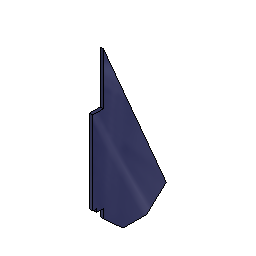
FIN_BUILD_1 (Autodesk Fusion 360 design; units mm, degrees)
Autodesk Fusion 360 part; units mm, degrees
note: some values were not read from the file. Set by a fixed rule: which sketch regions a step uses.
sketch "Sketch1" plane through (0, 0, 0) normal (0, 0, 1) x (1, 0, 0)
  circle A0 centre (0, 0) radius 29.75
  circle A1 centre (0, 0) radius 14.45
  circle A2 centre (0, 0) radius 18.45
  line L0 (0, 0) -> (0, 29.75) construction
  line L1 (-2, 23.3413) -> (-2, 18.3413)
  line L2 (-2, 23.3413) -> (-5, 23.3413)
  line L3 (-5, 23.3413) -> (-5, 17.7596)
  line L4 (2, 23.3413) -> (2, 18.3413)
  line L5 (2, 23.3413) -> (5, 23.3413)
  line L6 (5, 23.3413) -> (5, 17.7596)
  line L7 (-21.2141, -9.9386) -> (-16.884, -7.4386)
  line L8 (-21.2141, -9.9386) -> (-22.7141, -7.3405)
  line L9 (-22.7141, -7.3405) -> (-17.8802, -4.5497)
  line L10 (-19.2141, -13.4027) -> (-14.884, -10.9027)
  line L11 (-17.7141, -16.0008) -> (-12.8802, -13.2099)
  line L12 (-19.2141, -13.4027) -> (-17.7141, -16.0008)
  line L13 (19.2141, -13.4027) -> (14.884, -10.9027)
  line L14 (19.2141, -13.4027) -> (17.7141, -16.0008)
  line L15 (17.7141, -16.0008) -> (12.8802, -13.2099)
  line L16 (21.2141, -9.9386) -> (16.884, -7.4386)
  line L17 (22.7141, -7.3405) -> (17.8802, -4.5497)
  line L18 (21.2141, -9.9386) -> (22.7141, -7.3405)
  circle A3 centre (0, 0) radius 16.5
  circle A4 centre (0, 0) radius 31.8
  dimension "d1" = 59.5
  dimension "d77" = 28.9
  dimension "d78" = 36.9
  dimension "d80" = 5
  dimension "d81" = 3
  dimension "d84" = 360
  dimension "d85" = 33
  dimension "d127" = 63.6
  constraint coincident A0.centre A1.centre
  constraint concentric A0 A1
  constraint coincident A0 L0.end
  constraint vertical L0
  constraint vertical L1
  constraint coincident A2 L1.end
  constraint perpendicular L1 L2
  constraint coincident A2 L3.end
  constraint symmetric L0 L1.end L4.end
  constraint symmetric L0 L1.start L4.start
  constraint symmetric L0 L2.end L5.end
  constraint symmetric L0 L3.end L6.end
  constraint concentric A1 A3
  constraint parallel L1 L3
  constraint concentric A2 A4
  measures "d1" diameter of A0
  measures "d77" diameter of A1
  measures "d78" diameter of A2
  measures "d80" distance of L1.end L1.start
  measures "d81" distance of L1.start L2.end
  measures "d85" diameter of A3
  measures "d127" diameter of A4
sketch "Sketch11" plane through (0, 0, 0) normal (1, 0, 0) x (0, 1, 0)
  line L0 (18.45, 0) -> (-18.45, 0)
  line L1 (31.8, 0) -> (-31.8, 0)
  line L2 (23.3413, 4) -> (18.55, 4)
  line L3 (31.8, 0) -> (31.8, -1.744)
  line L4 (31.8, -1.744) -> (31.8, -11)
  line L5 (31.8, 119) -> (31.8, 109.8)
  line L6 (23.3413, 4) -> (23.5413, 4)
  line L7 (23.5413, 4) -> (23.5413, 0)
  line L8 (18.55, 109.8) -> (18.55, 4)
  line L9 (31.8, 109.8) -> (18.55, 109.8)
  line L10 (31.8, -11) -> (31.8, 176) construction
  line L11 (31.8, -11) -> (111.8, -11) construction
  line L12 (111.8, -11) -> (31.8, 176)
  line L13 (31.8, 176) -> (31.8, -34) construction
  line L14 (31.8, -34) -> (56.8, -34) construction
  line L15 (31.8, -34) -> (86.8, -34) construction
  line L16 (31.8, -11) -> (56.8, -34)
  line L17 (86.8, -34) -> (111.8, -11)
  line L18 (56.8, -34) -> (86.8, -34)
  line L19 (31.8, 176) -> (31.8, 119)
  point P0 (23.3413, 0)
  dimension "d128" = 4
  dimension "d135" = 11
  dimension "d148" = 0.2
  dimension "d165" = 187
  dimension "d166" = 80
  dimension "d167" = 210
  dimension "d168" = 25
  dimension "d169" = 55
  constraint coincident L1.start L3.start
  constraint perpendicular L1 L3
  constraint perpendicular L1 L4
  constraint horizontal L6
  constraint vertical L7
  constraint vertical L8
  constraint perpendicular L8 L9
  constraint parallel L4 L10
  constraint perpendicular L4 L11
  constraint perpendicular L11 L13
  constraint perpendicular L10 L14
  constraint perpendicular L13 L15
  constraint parallel L10 L19
  measures "d128" distance of P0 L2.start
  measures "d135" distance of L1 L4.end
  measures "d148" distance of L2.start L6.end
  measures "d165" distance of L4.end L10.end
  measures "d166" distance of L4.end L11.end
  measures "d167" distance of L10.end L13.end
  measures "d168" distance of L13.end L14.end
  measures "d169" distance of L13.end L15.end
extrude "Extrude16" add sketch "Sketch11" along normal blind 4
equation "d78 = 28.9 mm + 8 mm"
equation "d127 = 60 mm + ( 2 * 1.8 ) * 1 mm"
